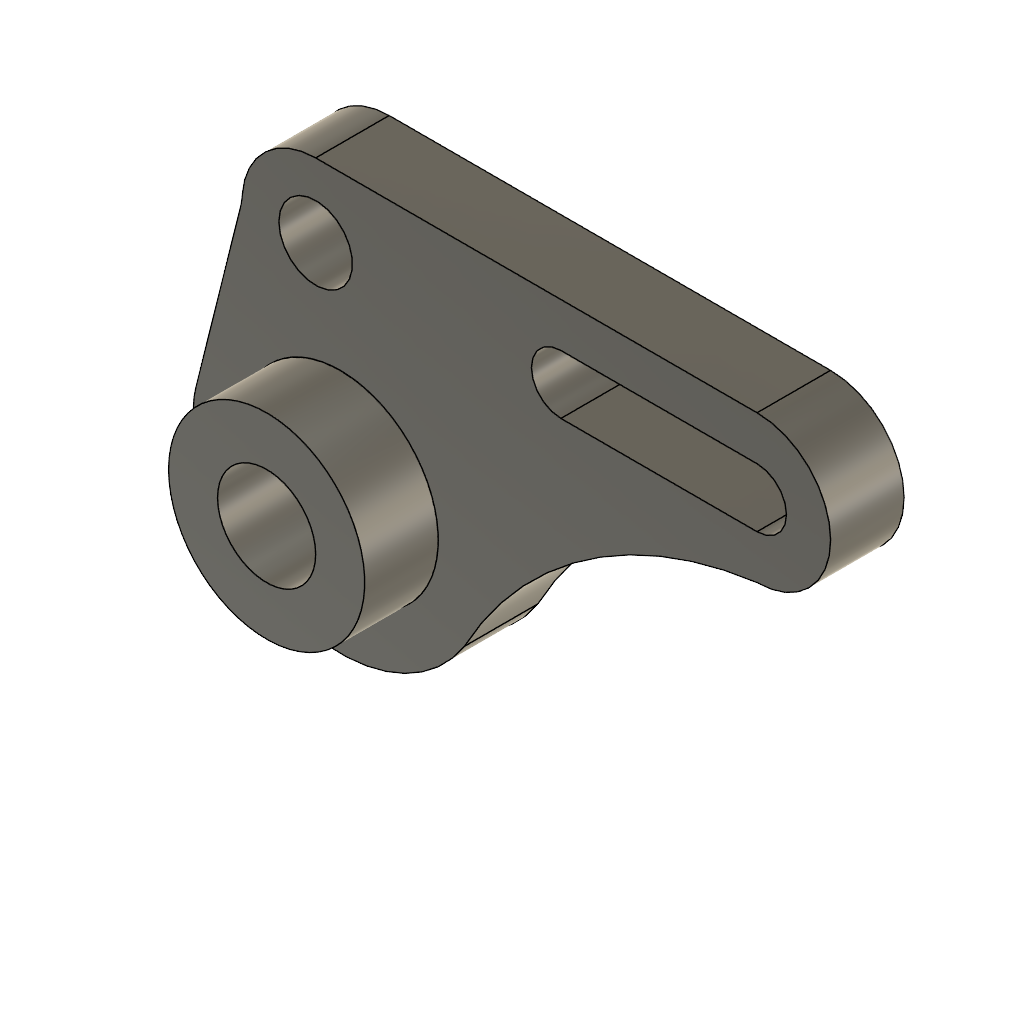
exercise 10 (Autodesk Fusion 360 design; units mm, degrees)
part number: 2026-10-06-22-14-11-788
Autodesk Fusion 360 part; units mm, degrees
sketch "Sketch1" plane through (0, 0, 0) normal (0, 1, 0) x (1, 0, 0)
  circle A0 centre (0, 0) radius 10
  circle A1 centre (0, 0) radius 20
  circle A2 centre (-5, -40) radius 7.5
  line L0 (85, -34) -> (45, -34)
  arc A3 (45, -34) -> (45, -46) centre (45, -40) ccw
  line L1 (45, -46) -> (85, -46)
  arc A4 (85, -46) -> (85, -34) centre (85, -40) ccw
  line L2 (85, -40) -> (45, -40) construction
  arc A5 (26.8508, 13.3803) -> (-29.843, 3.0652) centre (0, 0) ccw
  arc A6 (-19.9612, -41.0786) -> (-5, -55) centre (-5, -40) ccw
  arc A7 (85, -55) -> (85, -25) centre (85, -40) ccw
  line L3 (-20.3702, -38.5192) -> (-29.4736, -2.1054)
  arc A8 (-19.9612, -41.0786) -> (-20.3702, -38.5192) centre (-34.9223, -42.1572) ccw
  arc A9 (-29.843, 3.0652) -> (-29.4736, -2.1054) centre (-14.9215, 1.5326) ccw
  line L4 (-5, -55) -> (85, -55)
  arc A10 (25.3217, 16.0877) -> (85, -25) centre (95.2804, 53.8161) ccw
  point P0 (65, -40)
  dimension "d1" = 20
  dimension "d2" = 40
  dimension "d3" = 15
  dimension "d4" = 40
  dimension "d5" = 50
  dimension "d6" = 85
  dimension "d7" = 40
  dimension "d8" = 40
  dimension "d9" = 6
  dimension "d10" = 30
  dimension "d11" = 60
  dimension "d12" = 30
  dimension "d13" = 15
  dimension "d14" = 15
  constraint coincident A0.centre A1.centre
  constraint tangent L0 A3
  constraint tangent A3 L1
  constraint parallel L0 L1
  constraint tangent L1 A4
  constraint tangent L0 A4
  constraint horizontal L2
  constraint midpoint L2 P0
  constraint concentric A4 A7
  constraint concentric A1 A5
  constraint concentric A2 A6
  constraint tangent L3 A8
  constraint tangent A6 A8
  constraint tangent L3 A9
  constraint tangent A5 A9
  constraint tangent A7 L4
  constraint horizontal L4
  constraint coincident A5 A10.start
  constraint coincident A10 A5.start
  measures "d1" diameter of A0
  measures "d2" diameter of A1
  measures "d3" diameter of A2
  measures "d4" distance of A4.centre A3.centre
  measures "d5" horizontal distance of A2.centre A3.centre
  measures "d6" horizontal distance of A0.centre A4.centre
  measures "d7" vertical distance of A0.centre A2.centre
  measures "d8" vertical distance of A0.centre A4.centre
  measures "d9" radius of A3
  measures "d10" diameter of A7
  measures "d11" diameter of A5
  measures "d12" diameter of A6
  measures "d13" radius of A8
  measures "d14" radius of A9
extrude "Extrude1" add sketch "Sketch1" along normal blind 15 contours A5 A6 A7 L3 A8 A9 L4 A10 makes body 1
extrude "Extrude2" add sketch "Sketch1" against normal blind 15 separate body contours A1 makes body 2
